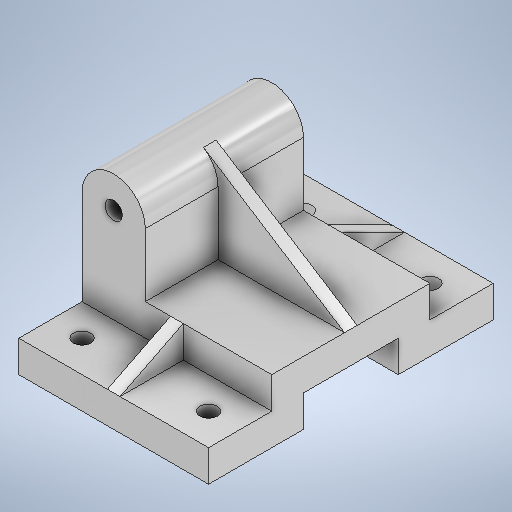
# Autodesk Inventor part: MMAE 232 Assignment 1_Part 1 - Dylan Tamras
Saved by Autodesk Inventor 2025.2 (Build 292293000, 293)
## iProperties
Created: 2025-02-02
Part Number: MMAE 232 Assignment 1_Part 1 - Dylan Tamras
Material: Generic
Document SubType Name: Modeling
Designer: Dylan
Density: 1 g/cm^3
Appearance: Default
Mass: 94.5733 g
Surface Area: 229.017 cm^2
Volume: 94.5733 cm^3
Author: VRK99-0110
Title: Mechanical Component - 01
Autodesk Inventor part; units mm, degrees
sketch "Sketch1" plane through (0, 0, 0) normal (0, 1, 0) x (-1, 0, 0)
  line L0 (0, 0) -> (60, 0)
  line L1 (60, 0) -> (60, -90)
  line L2 (60, -90) -> (0, -90)
  line L3 (0, -90) -> (0, 0)
  dimension "d0" = 60
  dimension "d1" = 90
  constraints: 8 end point, 3 perpendicular, 1 horizontal
  measures "d0" distance of L0.start L0.end
  measures "d1" distance of L0.end L1.end
extrude "Extrusion1" add sketch "Sketch1" along normal blind 10
sketch "Sketch2" plane through (0, 10, 0) normal (0, 1, 0) x (1, 0, 0)
  line L0 (0, 20) -> (-60, 20)
  line L1 (0, 70) -> (-60, 70)
  line L2 (-60, 70) -> (-60, 20)
  line L3 (0, 20) -> (0, 70)
  point P0 (0, 0)
  constraints: 8 end point, 1 parallel, 1 perpendicular
extrude "Extrusion2" add sketch "Sketch2" along normal blind 10
sketch "Sketch3" plane through (0, 0, 0) normal (0, -1, 0) x (1, 0, 0)
  line L0 (0, -30) -> (-60, -30)
  line L1 (-60, -30) -> (-60, -60)
  line L2 (0, -90) -> (0, -60)
  line L3 (0, -60) -> (-60, -60)
  line L4 (0, -60) -> (0, -30)
  dimension "d9" = 30
  constraints: 10 end point, 1 perpendicular
  measures "d9" distance of L0.end L1.end
extrude "Extrusion3" cut sketch "Sketch3" against normal blind 10
sketch "Sketch4" plane through (0, 10, 0) normal (0, 1, 0) x (1, 0, 0)
  circle A0 centre (-10, 10) radius 2.75
  circle A1 centre (-50, 10) radius 2.75
  dimension "d13" = 5.5
  dimension "d14" = 5.5
  constraints: 2 centre point
  measures "d13" diameter of A0
  measures "d14" diameter of A1
extrude "Extrusion4" cut sketch "Sketch4" against normal blind 10
ref_plane "Work Plane1" through (-30, 0, -90) normal (1, 0, 0) x (0, 0, -1)
sketch "Sketch5" plane through (-30, 0, -90) normal (1, 0, 0) x (0, 0, -1)
  line L0 (-70, 10) -> (-70, 20) projected
  line L1 (-90, 10) -> (-70, 10) projected
  line L2 (-70, 20) -> (-90, 10)
  line L3 (-90, 10) -> (-70, 10)
  line L4 (-70, 10) -> (-70, 20)
  point P0 (-90, 0)
  constraints: 6 end point, 1 collinear, 1 perpendicular
extrude "Extrusion5" add sketch "Sketch5" along normal mid plane 4
ref_plane "Work Plane2" through (-60, 0, -45) normal (0, 0, 1) x (1, 0, 0)
mirror "Mirror1" about plane through (-60, 0, -45) normal (0, 0, 1) of "Extrusion4", "Extrusion5"
sketch "Sketch6" plane through (0, 20, 0) normal (0, 1, 0) x (1, 0, 0)
  line L0 (-32, 70) -> (-60, 70) projected
  line L1 (-40, 20) -> (-40, 70)
  line L2 (-60, 70) -> (-40, 70)
  line L3 (-60, 70) -> (-60, 20)
  line L4 (-60, 20) -> (-40, 20)
  point P0 (0, 0)
  point P1 (0, 20)
  constraints: 8 end point, 2 perpendicular, 1 collinear, 1 point on line
extrude "Extrusion6" add sketch "Sketch6" along normal blind 30
fillet "Fillet1" radius 10 2 edges at (-40, 50, -45) (-60, 50, -45)
sketch "Sketch7" plane through (-32, 10, -70) normal (0, 0, -1) x (-1, 0, 0)
  arc A0 (28, 30) -> (8, 30) centre (18, 30) ccw projected
  circle A1 centre (18, 30) radius 2.75
  point P0 (-32, -10)
  dimension "d24" = 5.5
  constraints: 1 centre point, 1 coincident
  measures "d24" diameter of A1
extrude "Extrusion7" cut sketch "Sketch7" against normal blind 50
ref_plane "Work Plane3" through (-60, 10, -45) normal (0, 0, 1) x (1, 0, 0)
sketch "Sketch8" plane through (-60, 10, -45) normal (0, 0, 1) x (1, 0, 0)
  line L0 (32, 10) -> (60, 10) projected
  line L1 (60, 10) -> (15.3735, 38.4336)
  arc A0 (20, 30) -> (0, 30) centre (10, 30) ccw projected
  line L2 (15.3735, 38.4336) -> (15.3735, 10)
  line L3 (15.3735, 10) -> (60, 10)
  point P0 (60, -10)
  constraints: 6 end point, 1 perpendicular, 1 point on circle, 1 tangent, 1 vertical
extrude "Extrusion8" add sketch "Sketch8" along normal mid plane 4
body "Solid1"
